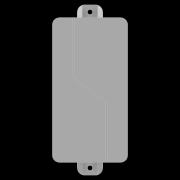
# Autodesk Inventor part: fishman-modern6
Saved by Autodesk Inventor 2020 (Build 240168000, 168)
## iProperties
Created: 2020-01-01
Part Number: fishman-modern6
Material: Generic
Document SubType Name: Modeling
Designer: valer
Density: 1 g/cm^3
Appearance: Default
Author: valer
Autodesk Inventor part; units mm, degrees
ref_plane "YZ Plane" through (0, 0, 0) normal (1, 0, 0) x (0, 1, 0)
ref_plane "XZ Plane" through (0, 0, 0) normal (0, 1, 0) x (-1, 0, 0)
sketch "FishmanModern6" plane through (0, 0, 0) normal (0, 0, 1) x (1, 0, 0)
  line L0 (-18.8087, 42.4942) -> (18.8087, 42.4942) construction
  line L1 (18.8087, 42.4942) -> (18.8087, -42.4942) construction
  line L2 (18.8087, -42.4942) -> (-18.8087, -42.4942) construction
  line L3 (-18.8087, -42.4942) -> (-18.8087, 42.4942) construction
  line L4 (-18.8087, 0) -> (18.8087, 0) construction
  line L5 (0, 42.4942) -> (0, -42.4942) construction
  line L6 (0, 38.9001) -> (0, -38.9001) construction
  circle A0 centre (0, 38.9001) radius 1.27
  circle A1 centre (0, -38.9001) radius 1.27
  line L7 (-6.35, 42.4942) -> (6.35, 42.4942)
  line L8 (6.35, 42.4942) -> (6.35, 36.1442)
  line L9 (6.35, -42.4942) -> (-6.35, -42.4942)
  line L10 (-6.35, -42.4942) -> (-6.35, -36.1442)
  line L11 (-18.8087, 36.1442) -> (18.8087, 36.1442)
  line L12 (18.8087, 36.1442) -> (18.8087, -36.1442)
  line L13 (18.8087, -36.1442) -> (-18.8087, -36.1442)
  line L14 (-18.8087, -36.1442) -> (-18.8087, 36.1442)
  line L15 (-6.35, 36.1442) -> (-6.35, 42.4942)
  line L16 (6.35, 36.1442) -> (6.35, -36.1442) construction
  line L17 (-6.35, -36.1442) -> (-6.35, 36.1442) construction
  line L18 (6.35, -36.1442) -> (6.35, -42.4942)
  point P0 (0, 0)
  point P1 (0, 0)
  point P2 (0, 36.1442)
  point P3 (0, 0)
  dimension "d1" = 84.9884
  dimension "d2" = 37.6174
  dimension "d3" = 77.8002
  dimension "d4" = 2.54
  dimension "d5" = 12.7
  dimension "d6" = 6.35
  dimension "d7" = 6.35
  dimension "d132" = 72.2884
  constraints: 38 end point, 14 parallel, 9 midpoint, 7 point on line, 5 perpendicular, 3 coincident, 3 horizontal, 2 centre point, 1 collinear, 1 equal radius, 1 vertical
  measures "d1" distance of L2.end L0.start
  measures "d2" distance of L0.start L0.end
  measures "d3" distance of L6.start L6.end
  measures "d4" diameter of A0
  measures "d5" distance of L7.end L7.start
  measures "d6" distance between parallel lines of L0 L11
  measures "d7" distance between parallel lines of L2 L13
  measures "d132" distance of L13.end L11.start
extrude "FishmanModern6Feature" add sketch "FishmanModern6" along normal blind 18.0086 contours L11 L12 L13 L14
fillet "FishmanModern6FilletsFeature" radius 3.6576 4 edges at (-18.8087, 36.1442, 9.0043) (-18.8087, -36.1442, 9.0043) (18.8087, -36.1442, 9.0043) (18.8087, 36.1442, 9.0043)
ref_plane "FishmanModern6LegPlane" through (0, 0, -7.0866) normal (0, 0, -1) x (-1, 0, 0)
ref_plane "FishmanModern6SepPlane" through (0, 0, -4.5974) normal (0, 0, -1) x (-1, 0, 0)
sketch "FishmanModern6Legs" plane through (0, 0, -7.0866) normal (0, 0, -1) x (-1, 0, 0)
  line L0 (-6.35, 42.4942) -> (-6.35, 36.1442) projected
  line L1 (6.35, 42.4942) -> (-6.35, 42.4942) projected
  line L2 (6.35, 36.1442) -> (6.35, 42.4942) projected
  circle A0 centre (0, 38.9001) radius 1.27 projected
  line L3 (-6.35, -36.1442) -> (-6.35, -42.4942) projected
  line L4 (6.35, -42.4942) -> (6.35, -36.1442) projected
  line L5 (-6.35, -42.4942) -> (6.35, -42.4942) projected
  circle A1 centre (0, -38.9001) radius 1.27 projected
  line L6 (-6.35, 36.1442) -> (6.35, 36.1442)
  line L7 (-6.35, -36.1442) -> (6.35, -36.1442)
  line L8 (-6.35, 36.1442) -> (6.35, 36.1442)
  line L9 (6.35, 36.1442) -> (6.35, 34.3662)
  line L10 (6.35, 34.3662) -> (-6.35, 34.3662)
  line L11 (-6.35, 34.3662) -> (-6.35, 36.1442)
  line L12 (-6.35, -36.1442) -> (6.35, -36.1442)
  line L13 (6.35, -36.1442) -> (6.35, -34.3662)
  line L14 (6.35, -34.3662) -> (-6.35, -34.3662)
  line L15 (-6.35, -34.3662) -> (-6.35, -36.1442)
  point P0 (0, 0)
  dimension "d120" = 1.778
  constraints: 20 end point, 4 horizontal, 4 parallel, 3 collinear, 2 perpendicular
  measures "d120" distance of L10.end L0.end
extrude "FishmanModern6LegsFeature" add sketch "FishmanModern6Legs" against normal up to surface (2.4892 mm away)
sketch "FishmanModern6LegLoft1" plane through (-6.35, 36.1442, -4.5974) normal (0, 0, 1) x (1, 0, 0)
  line L0 (10.16, 6.35) -> (10.16, 0)
  line L1 (10.16, 0) -> (12.7, 0)
  line L2 (12.7, 0) -> (12.7, 6.35)
  line L3 (-8.8011, -72.2884) -> (21.5011, -72.2884) construction
  line L4 (-8.8011, -72.2884) -> (21.5011, -72.2884) construction
  line L5 (21.5011, 0) -> (-8.8011, 0) construction
  line L6 (12.7, 6.35) -> (10.16, 6.35)
  line L7 (12.7, -1.778) -> (12.7, 6.35) construction
  line L8 (12.7, 6.35) -> (0, 6.35) construction
  point P0 (6.35, -36.1442)
  dimension "d121" = 2.54
  constraints: 8 end point, 3 collinear, 1 parallel
  measures "d121" distance of L2.end L0.start
sketch "FishmanModern6LegLoft2" plane through (-15.1511, 36.1442, 0) normal (0, 1, 0) x (1, 0, 0)
  line L0 (18.9611, 4.5974) -> (21.5011, 4.5974) projected
  line L1 (21.5011, 4.5974) -> (21.5011, -2.54)
  line L2 (21.5011, -2.54) -> (18.9611, -2.54)
  line L3 (18.9611, -2.54) -> (18.9611, 4.5974)
  line L4 (30.3022, 0) -> (0, 0) projected
  point P0 (15.1511, 0)
  point P1 (11.3411, 4.5974)
  point P2 (8.8011, 4.5974)
  dimension "d115" = 2.54
  constraints: 6 end point, 2 perpendicular, 1 vertical
  measures "d115" distance between parallel lines of L4 L2
loft "FishmanModern6LegJoinFeature" add profiles "FishmanModern6LegLoft1", "FishmanModern6LegLoft2" separate body
mirror "FishmanModern6Loft1Feature" about plane through (0, 0, 0) normal (1, 0, 0) bodies 2
mirror "FishmanModern6Loft2Feature" about plane through (0, 0, 0) normal (0, 1, 0) of "FishmanModern6LegJoinFeature", "FishmanModern6Loft1Feature" bodies 2
sketch "FishmanModern6Join" plane through (-6.35, 42.4942, -4.5974) normal (0, 0, 1) x (1, 0, 0)
  line L0 (0, -8.128) -> (12.7, -8.128) projected
  line L1 (0, -6.35) -> (2.54, -6.35) projected
  line L2 (0, -8.128) -> (12.7, -8.128)
  line L3 (12.7, -8.128) -> (12.7, -6.35)
  line L4 (12.7, -6.35) -> (0, -6.35)
  line L5 (0, -6.35) -> (0, -8.128)
  line L6 (12.7, -8.128) -> (12.7, 0) projected
  line L7 (12.7, -76.8604) -> (0, -76.8604) projected
  line L8 (12.7, -78.6384) -> (0, -78.6384)
  line L9 (0, -78.6384) -> (0, -76.8604)
  line L10 (0, -76.8604) -> (12.7, -76.8604)
  line L11 (12.7, -76.8604) -> (12.7, -78.6384)
  line L12 (0, -78.6384) -> (2.54, -78.6384) projected
  line L13 (0, -76.8604) -> (0, -84.9884) projected
  line L14 (12.7, -84.9884) -> (12.7, -76.8604) projected
  point P0 (6.35, -42.4942)
  point P1 (0, -76.8604)
  constraints: 16 end point, 6 collinear, 4 parallel, 2 horizontal, 2 perpendicular
extrude "FishmanModern6JonFeature" add sketch "FishmanModern6Join" along normal up to surface (4.5974 mm away) bodies 1
combine bodies "FishmanModern6CombineFeature" operation type add bodies to combine 1 2
fillet "FishmanModern6LegFilletsFeatures" radius 3.6576 4 edges at (6.35, 42.4942, -5.842) (-6.35, 42.4942, -5.842) (-6.35, -42.4942, -5.842) (6.35, -42.4942, -5.842)
sketch "FishmanModern6IndentFeature" plane through (0, 0, 18.0086) normal (0, 0, 1) x (1, 0, 0)
  line L0 (-6.6675, 4.6686) -> (6.6675, -4.6686)
  line L1 (-8.2272, 7.6648) -> (-8.2272, 36.1442)
  line L2 (8.2272, -7.6648) -> (8.2272, -36.1442)
  arc A0 (8.2272, -7.6648) -> (6.6675, -4.6686) centre (4.5696, -7.6648) ccw
  arc A1 (-8.2272, 7.6648) -> (-6.6675, 4.6686) centre (-4.5696, 7.6648) ccw
  line L3 (-18.8087, 32.4866) -> (-18.8087, -32.4866) construction
  line L4 (18.8087, -32.4866) -> (18.8087, 32.4866) construction
  line L5 (-15.1511, -36.1442) -> (15.1511, -36.1442) construction
  line L6 (15.1511, 36.1442) -> (-15.1511, 36.1442) construction
  line L7 (7.8462, -36.1442) -> (7.8462, -7.6648)
  arc A2 (7.8462, -7.6648) -> (6.449, -4.9807) centre (4.5696, -7.6648) ccw
  line L8 (6.449, -4.9807) -> (-6.886, 4.3565)
  arc A3 (-8.6082, 7.6648) -> (-6.886, 4.3565) centre (-4.5696, 7.6648) ccw
  line L9 (-8.6082, 7.6648) -> (-8.6082, 36.1442)
  line L10 (8.6082, -36.1442) -> (8.6082, -7.6648)
  arc A4 (8.6082, -7.6648) -> (6.886, -4.3565) centre (4.5696, -7.6648) ccw
  line L11 (6.886, -4.3565) -> (-6.449, 4.9807)
  arc A5 (-7.8462, 7.6648) -> (-6.449, 4.9807) centre (-4.5696, 7.6648) ccw
  line L12 (-7.8462, 7.6648) -> (-7.8462, 36.1442)
  line L13 (7.8462, -36.1442) -> (8.6082, -36.1442)
  line L14 (-8.6082, 36.1442) -> (-7.8462, 36.1442)
  point P0 (0, 0)
  point P1 (0, 0)
  dimension "d125" = 3.6576
  dimension "d126" = 125
  dimension "d127" = 13.335
  dimension "d128" = 0.381
  dimension "d129" = 0.381
  constraints: 22 end point, 12 point on circle, 6 centre point, 4 tangent, 2 collinear, 2 parallel, 2 point on line, 1 coincident, 1 equal radius, 1 horizontal, 1 midpoint, 1 perpendicular, 8 other
  measures "d125" radius of A0
  measures "d126" angle of L1 L0
  measures "d127" horizontal distance of L0.start L0.end
  measures "d128" distance between parallel lines of L2 L7
  measures "d129" distance between parallel lines of L2 L10
extrude "Extrusion8" cut sketch "FishmanModern6IndentFeature" against normal blind 0.762 bodies 1
equation "\"d7\" = d6"
body "Solid1"
